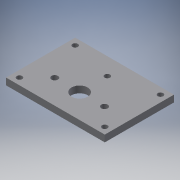
# Autodesk Inventor part: pumpHead
Saved by Autodesk Inventor 2017 (Build 210142000, 142)
## iProperties
Created: 2016-11-08
Part Number: pumpHead
Material: Generic
Document SubType Name: Modeling
Designer: Camilo
Density: 1 g/cm^3
Appearance: Default
Author: Camilo
Autodesk Inventor part; units mm, degrees
ref_plane "YZ Plane" through (0, 0, 0) normal (1, 0, 0) x (0, 1, 0)
ref_plane "XZ Plane" through (0, 0, 0) normal (0, 1, 0) x (-1, 0, 0)
ref_plane "XY Plane" through (0, 0, 0) normal (0, 0, 1) x (1, 0, 0)
sketch "Sketch1" plane through (0, 0, 0) normal (0, 0, 1) x (1, 0, 0)
  line L0 (-31.7, -20.7) -> (31.7, -20.7) construction
  line L1 (31.7, -20.7) -> (31.7, 20.7) construction
  line L2 (31.7, 20.7) -> (-31.7, 20.7) construction
  line L3 (-31.7, 20.7) -> (-31.7, -20.7) construction
  line L4 (-31.7, -20.7) -> (31.7, 20.7) construction
  line L5 (31.7, -20.7) -> (-31.7, 20.7) construction
  circle A0 centre (-31.7, 20.7) radius 2
  circle A1 centre (31.7, 20.7) radius 2
  circle A2 centre (31.7, -20.7) radius 2
  circle A3 centre (-31.7, -20.7) radius 2
  circle A4 centre (0, 12.9) radius 2
  circle A5 centre (0, -7.7) radius 6
  circle A6 centre (-18.5, -7.7) radius 2.4
  circle A7 centre (18.5, -7.7) radius 2.4
  line L6 (0, 20.7) -> (0, -20.7) construction
  line L7 (36.7, -25.7) -> (-36.7, -25.7)
  line L8 (-36.7, -25.7) -> (-36.7, 25.7)
  line L9 (-36.7, 25.7) -> (36.7, 25.7)
  line L10 (36.7, 25.7) -> (36.7, -25.7)
  point P0 (0, 0)
  dimension "d0" = 63.4
  dimension "d1" = 41.4
  dimension "d2" = 4
  dimension "d3" = 31.7
  dimension "d4" = 7.8
  dimension "d5" = 31.7
  dimension "d6" = 13
  dimension "d7" = 12
  dimension "d8" = 18.5
  dimension "d9" = 0
  dimension "d10" = 4.8
  dimension "d11" = 5
  constraints: 22 end point, 8 centre point, 4 coincident, 4 equal radius, 4 midpoint, 4 parallel, 2 perpendicular, 1 horizontal, 4 other
  measures "d0" distance of L0.start L0.end
  measures "d1" distance of L1.end L0.end
  measures "d2" diameter of A0
  measures "d3" horizontal distance of L1.end A4.centre
  measures "d4" vertical distance of L1.end A4.centre
  measures "d5" horizontal distance of L0.start A5.centre
  measures "d6" vertical distance of L0.start A5.centre
  measures "d7" diameter of A5
  measures "d8" distance of A5.centre A6.centre
  measures "d9" vertical distance of A5.centre A6.centre
  measures "d10" diameter of A6
  measures "d11" distance from line of L8 A0.centre
extrude "Extrusion1" add sketch "Sketch1" along normal blind 5
body "Solid1"
